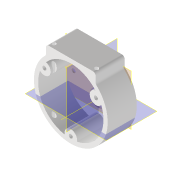
# Autodesk Inventor part: Pump_Base_Motor_new
Saved by Autodesk Inventor 2022.5 (Build 265521000, 521)
## iProperties
Created: 2023-11-14
Part Number: Pump_Base_Motor_new
Material: Generisch
Document SubType Name: Modeling
Designer: diederichbenedict
Density: 1 g/cm^3
Appearance: Vorgabe
Author: diederichbenedict
Autodesk Inventor part; units mm, degrees
ref_plane "YZ Plane" through (0, 0, 0) normal (1, 0, 0) x (0, 1, 0)
ref_plane "XZ Plane" through (0, 0, 0) normal (0, 1, 0) x (-1, 0, 0)
ref_plane "XY Plane" through (0, 0, 0) normal (0, 0, 1) x (1, 0, 0)
ref_plane "Arbeitsebene1" through (0, 0, 0) normal (0, 0, 1) x (1, 0, 0)
sketch "Skizze1" plane through (0, 0, 0) normal (0, 0, 1) x (1, 0, 0)
  arc A0 (-13.5554, 10.695) -> (13.5554, 10.695) centre (0, 14.195) ccw projected
  arc A1 (19.6, 14.195) -> (15.4, 14.195) centre (17.5, 14.195) ccw projected
  circle A2 centre (-17.5, 14.195) radius 2.1 projected
  arc A3 (4.55, 6.195) -> (-4.55, 6.195) centre (0, 6.195) ccw projected
  circle A4 centre (0, 14.195) radius 26
  circle A5 centre (-17.5, 14.195) radius 1.4
  circle A6 centre (17.5, 14.195) radius 1.4
  circle A7 centre (0, 6.195) radius 6
  point P0 (0, 0)
  dimension "d0" = 52
  dimension "d1" = 2.8
  dimension "d2" = 2.8
  dimension "d3" = 12
  constraints: 4 centre point, 4 coincident
  measures "d0" diameter of A4
  measures "d1" diameter of A5
  measures "d2" diameter of A6
  measures "d3" diameter of A7
extrude "Extrusion1" add sketch "Skizze1" against normal blind 1 contours A2 | A4
sketch "Skizze2" plane through (0, 14.195, 0) normal (0, 0, 1) x (1, 0, 0)
  circle A0 centre (0, 0) radius 26 projected
  circle A1 centre (0, -8) radius 6 projected
  circle A2 centre (17.5, 0) radius 1.4 projected
  arc A3 (14, 0) -> (-14, 0) centre (0, 0) ccw projected
  circle A4 centre (0, 0) radius 14 projected
  line L0 (-13.5554, -3.5) -> (-17.5, -3.5) projected
  arc A5 (-17.5, 3.5) -> (-17.5, -3.5) centre (-17.5, 0) ccw projected
  line L1 (-17.5, 3.5) -> (-13.5554, 3.5) projected
  line L2 (-8.75, 18.5) -> (-8.75, 10.9287) projected
  line L3 (8.75, 18.5) -> (-8.75, 18.5) projected
  line L4 (8.75, 18.5) -> (8.75, 10.9287) projected
  circle A6 centre (0, 0) radius 23
  circle A7 centre (-17.5, 0) radius 1.4
  point P0 (0, -14.195)
  dimension "d6" = 3
  dimension "d9" = 2.8
  constraints: 2 centre point, 1 coincident
  measures "d6" radial gap between concentric circles of A0 A6
  measures "d9" diameter of A7
ref_plane "Arbeitsebene2" through (-14.0001, 0.1949, 19.5) normal (0, 0, 1) x (1, 0, 0)
extrude "Extrusion2" add sketch "Skizze2" along normal up to surface (19.5 mm away) contours A0
ref_plane "Arbeitsebene4" through (0, 6.195, -1) normal (0, -1, 0) x (0, 0, 1)
ref_plane "Arbeitsebene3" through (0, 25.1237, 0) normal (-1, 0, 0) x (0, 0, 1)
sketch "Skizze6" plane through (0, 14.195, 0) normal (0, 0, 1) x (1, 0, 0)
  circle A0 centre (14.9794, -15.0186) radius 1.6
  circle A1 centre (-15.0206, -15.0185) radius 1.6
  circle A2 centre (-15.0206, 14.9815) radius 1.6
  circle A3 centre (14.9794, 14.9814) radius 1.6
  circle A4 centre (0, 0) radius 23 projected
  circle A5 centre (14.9794, 14.9814) radius 4.6
  circle A6 centre (14.9794, -15.0186) radius 4.6
  circle A7 centre (-15.0206, -15.0185) radius 4.6
  circle A8 centre (-15.0206, 14.9815) radius 4.6
  point P0 (12.864, 19.0661)
  point P1 (19.0644, 12.8665)
  point P2 (-12.8819, 19.054)
  point P3 (-19.0876, 12.8322)
  point P4 (-19.0766, -12.8485)
  point P5 (-12.8511, -19.0748)
  dimension "d42" = 3
  dimension "d43" = 3
  dimension "d44" = 3
  dimension "d45" = 3
  constraints: 8 centre point, 8 other
  measures "d42" radial gap between concentric circles of A3 A5
  measures "d43" radial gap between concentric circles of A0 A6
  measures "d44" radial gap between concentric circles of A1 A7
  measures "d45" radial gap between concentric circles of A2 A8
extrude "Extrusion4" add sketch "Skizze6" along normal up to surface (19.5 mm away) contours A5 A4 | A6 A4 | A4 A6 | A8 A4 | A4 A7 picked at (17.5763, 14.0989) picked at (-17.6054, 14.0788) picked at (-17.5961, -14.1029)
sketch "Skizze7" plane through (0, 14.195, 19.5) normal (0, 0, 1) x (1, 0, 0)
  arc A0 (-12.8511, -19.0748) -> (12.8329, -19.0871) centre (0, 0) ccw projected
  circle A1 centre (0, 0) radius 26 projected
  circle A2 centre (0, 0) radius 26 projected
  line L0 (-17.5, 19.2289) -> (-17.5, 26)
  line L1 (-17.5, 26) -> (17.5, 26)
  line L2 (17.5, 26) -> (17.5, 19.2289)
  circle A3 centre (0, 0) radius 26 projected
  arc A4 (-12.8511, -19.0748) -> (-19.0766, -12.8485) centre (-15.0206, -15.0185) ccw projected
  arc A5 (-19.0876, 12.8322) -> (-19.0766, -12.8485) centre (0, 0) ccw projected
  arc A6 (-19.0876, 12.8322) -> (-12.8819, 19.054) centre (-15.0206, 14.9815) ccw projected
  arc A7 (12.864, 19.0661) -> (-12.8819, 19.054) centre (0, 0) ccw projected
  arc A8 (12.864, 19.0661) -> (19.0644, 12.8665) centre (14.9794, 14.9814) ccw projected
  arc A9 (19.0535, -12.8827) -> (19.0644, 12.8665) centre (0, 0) ccw projected
  arc A10 (19.0535, -12.8827) -> (12.8329, -19.0871) centre (14.9794, -15.0186) ccw projected
  point P0 (0, -14.195)
  point P1 (0, 26)
  dimension "d28" = 35
  constraints: 6 end point, 2 perpendicular, 2 point on circle, 1 tangent, 1 vertical
  measures "d28" distance between parallel lines of L2 L0
extrude "Extrusion5" add sketch "Skizze7" against normal up to surface (20.5 mm away) contours A1 L1 L2 | L0 L1 A1
fillet "Rundung1" radius 2 4 edges at (-17.5, 33.4239, 9.25) (-17.5, 40.195, 9.25) (17.5, 33.4239, 9.25) (17.5, 40.195, 9.25)
sketch "Skizze8" plane through (-15.5, 40.195, 19.5) normal (0, 1, 0) x (1, 0, 0)
  line L0 (30.5, 38) -> (0.5, 38)
  line L1 (0.5, 38) -> (0.5, 3)
  line L2 (0.5, 3) -> (30.5, 3)
  line L3 (30.5, 3) -> (30.5, 38)
  line L4 (9.5, 20.5) -> (21.5, 20.5) projected
  line L5 (30.5, 38) -> (0.5, 3) construction
  line L6 (0.5, 38) -> (30.5, 3) construction
  point P0 (15.5, 19.5)
  point P1 (15.5, 20.5)
  point P2 (0.5, 3)
  dimension "d33" = 30
  dimension "d34" = 35
  constraints: 12 end point, 3 midpoint, 2 coincident, 2 parallel, 1 horizontal, 1 perpendicular
  measures "d33" distance of L2.end L1.end
  measures "d34" distance of L1.end L0.end
hole "Bohrung1" at (-15, 40.195, 16.5) at (15, 40.195, 16.5) direction (0, -1, 0) diameter 2.8 end through all
sketch "Skizze9" plane through (-15.5, 40.195, 19.5) normal (0, 0, 1) x (1, 0, 0)
  arc A0 (-2.6071, -7.3417) -> (33.6071, -7.3417) centre (15.5, -26) ccw
  arc A1 (33, -2) -> (31, 0) centre (31, -2) ccw projected
  line L0 (31, 0) -> (0, 0) projected
  arc A2 (0, 0) -> (-2, -2) centre (0, -2) ccw projected
  line L1 (-2, -2) -> (-2, -5.9065) projected
  arc A3 (-2.6071, -7.3417) -> (-2, -5.9065) centre (-4, -5.9065) ccw projected
  arc A4 (-2.6071, -7.3417) -> (33.6071, -7.3417) centre (15.5, -26) ccw projected
  arc A5 (33, -5.9065) -> (33.6071, -7.3417) centre (35, -5.9065) ccw projected
  line L2 (33, -5.9065) -> (33, -2) projected
  circle A6 centre (0.4794, -11.0185) radius 1.6 projected
  circle A7 centre (30.4794, -41.0186) radius 1.6 projected
  circle A8 centre (30.4794, -11.0186) radius 1.6 projected
  circle A9 centre (0.4794, -41.0185) radius 1.6 projected
  arc A10 (2.6489, -45.0748) -> (28.3329, -45.0871) centre (15.5, -26) ccw projected
  arc A11 (2.6489, -45.0748) -> (-3.5766, -38.8485) centre (0.4794, -41.0185) ccw projected
  arc A12 (-3.5876, -13.1678) -> (-3.5766, -38.8485) centre (15.5, -26) ccw projected
  arc A13 (-3.5876, -13.1678) -> (2.6181, -6.946) centre (0.4794, -11.0185) ccw projected
  arc A14 (28.364, -6.9339) -> (2.6181, -6.946) centre (15.5, -26) ccw projected
  arc A15 (28.364, -6.9339) -> (34.5644, -13.1335) centre (30.4794, -11.0186) ccw projected
  arc A16 (34.5535, -38.8827) -> (34.5644, -13.1335) centre (15.5, -26) ccw projected
  arc A17 (34.5535, -38.8827) -> (28.3329, -45.0871) centre (30.4794, -41.0186) ccw projected
  circle A18 centre (30.4794, -41.0186) radius 1.6 projected
  circle A19 centre (0.4794, -41.0185) radius 1.6 projected
  circle A20 centre (30.4794, -11.0186) radius 1.6 projected
  point P0 (15.5, -40.195)
  constraints: 4 coincident, 2 point on circle, 1 centre point, 4 other
hole "Bohrung2" at (14.9794, -0.8236, 19.5) at (-15.0206, -0.8235, 19.5) at (-15.0206, 29.1765, 19.5) at (14.9794, 29.1764, 19.5) direction (0, 0, -1) diameter 2.8 depth 30 tip angle 118 counterbore diameter 6.5 counterbore depth 3.5
